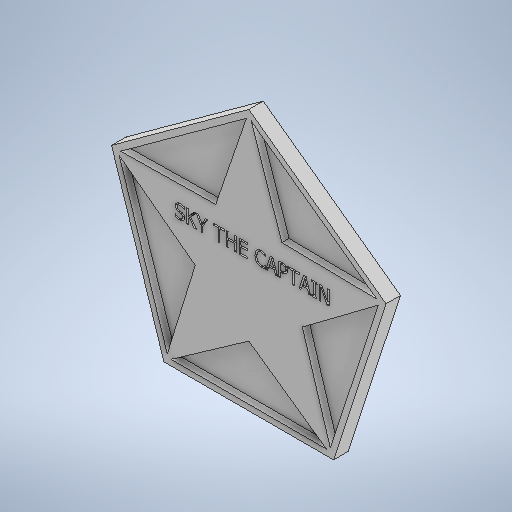
# Autodesk Inventor part: cad@24
Saved by Autodesk Inventor 2025.2 (Build 292293000, 293)
## iProperties
Created: 2025-03-15
Part Number: cad@24
Material: Generic
Document SubType Name: Modeling
Designer: spars
Density: 1 g/cm^3
Appearance: Default
Author: spars
Autodesk Inventor part; units mm, degrees
note: some values were not read from the file. Chosen so that the rebuilt part matches the saved one: direction of "Emboss1".
ref_plane "YZ Plane" through (0, 0, 0) normal (1, 0, 0) x (0, 1, 0)
ref_plane "XZ Plane" through (0, 0, 0) normal (0, 1, 0) x (-1, 0, 0)
ref_plane "XY Plane" through (0, 0, 0) normal (0, 0, 1) x (1, 0, 0)
sketch "Sketch1" plane through (0, 0, 0) normal (0, 0, 1) x (1, 0, 0)
  circle A0 centre (0, 0) radius 10 construction
  line L0 (0, 10) -> (9.5106, 3.0902)
  line L1 (9.5106, 3.0902) -> (5.8779, -8.0902)
  line L2 (5.8779, -8.0902) -> (-5.8779, -8.0902)
  line L3 (-5.8779, -8.0902) -> (-9.5106, 3.0902)
  line L4 (-9.5106, 3.0902) -> (0, 10)
  line L5 (0, 0) -> (0, -3.9)
  dimension "d0" = 20
  dimension "d1" = 3.9
  constraints: 12 end point, 2 coincident, 1 vertical, 1 vertical alignment, 13 other
  measures "d1" distance of L5.start L5.end
extrude "Extrusion1" add sketch "Sketch1" along normal blind 1
sketch "Sketch2" plane through (0, 0, 1) normal (0, 0, 1) x (1, 0, 0)
  line L0 (0.1618, 9.388) -> (8.8785, 3.0549)
  line L1 (8.9785, 2.7472) -> (5.649, -7.5)
  line L2 (5.3872, -7.6902) -> (-5.3872, -7.6902)
  line L3 (-5.649, -7.5) -> (-8.9785, 2.7472)
  line L4 (-8.8785, 3.0549) -> (-0.1618, 9.388)
  line L5 (-5.8779, -8.0902) -> (5.8779, -8.0902) projected
  line L6 (5.8779, -8.0902) -> (9.5106, 3.0902) projected
  line L7 (0, 10) -> (-9.5106, 3.0902) projected
  line L8 (9.5106, 3.0902) -> (0, 10) projected
  line L9 (-9.5106, 3.0902) -> (-5.8779, -8.0902) projected
  line L10 (0, 0) -> (0, -3.9)
  line L11 (0, -3.9) -> (-5.3872, -7.6902)
  line L12 (0, -3.9) -> (5.3872, -7.6902)
  line L13 (3.7091, -1.2052) -> (5.649, -7.5)
  line L14 (3.7091, -1.2052) -> (8.9785, 2.7472)
  line L15 (2.2924, 3.1552) -> (8.8785, 3.0549)
  line L16 (2.2924, 3.1552) -> (0.1618, 9.388)
  line L17 (-2.2924, 3.1552) -> (-0.1618, 9.388)
  line L18 (-2.2924, 3.1552) -> (-8.8785, 3.0549)
  line L19 (-3.7091, -1.2052) -> (-8.9785, 2.7472)
  line L20 (-3.7091, -1.2052) -> (-5.649, -7.5)
  point P0 (0, 9.5056)
  point P1 (9.0403, 2.9374)
  point P2 (5.5872, -7.6902)
  point P3 (-5.5872, -7.6902)
  point P4 (-9.0403, 2.9374)
  point P5 (8.8785, 3.0549)
  point P6 (-8.9785, 2.7472)
  dimension "d4" = 0.4
  dimension "d5" = 0.4
  dimension "d6" = 0.4
  dimension "d7" = 0.4
  dimension "d8" = 0.4
  dimension "d9" = 0.2
  dimension "d10" = 0.2
  dimension "d11" = 0.2
  dimension "d12" = 0.2
  dimension "d13" = 0.2
  dimension "d14" = 0.2
  dimension "d15" = 0.2
  dimension "d16" = 0.2
  dimension "d17" = 0.2
  dimension "d18" = 0.2
  dimension "d19" = 3.9
  dimension "d22" = 360
  constraints: 32 end point, 10 point on line, 1 coincident, 1 vertical, 37 other
  measures "d4" distance between parallel lines of L5 L2
  measures "d5" distance between parallel lines of L6 L1
  measures "d6" distance between parallel lines of L4 L7
  measures "d7" distance between parallel lines of L0 L8
  measures "d8" distance between parallel lines of L9 L3
  measures "d9" distance of L3.end point (-9.04, 2.937)
  measures "d10" distance of L4.start point (-9.04, 2.937)
  measures "d11" distance of L4.end point (0, 9.506)
  measures "d12" distance of L0.start point (0, 9.506)
  measures "d13" distance of L0.end point (9.04, 2.937)
  measures "d14" distance of L1.start point (9.04, 2.937)
  measures "d15" distance of L2.start point (5.587, -7.69)
  measures "d16" distance of L1.end point (5.587, -7.69)
  measures "d17" distance of L3.start point (-5.587, -7.69)
  measures "d18" distance of L2.end point (-5.587, -7.69)
  measures "d19" distance of L10.start L10.end
extrude "Extrusion2" cut sketch "Sketch2" against normal blind 0.5 contours L0 L15 L16 | L1 L13 L14 | L2 L11 L12 | L3 L19 L20 | L4 L17 L18
sketch "Sketch3" plane through (0, 0, 1) normal (0, 0, 1) x (1, 0, 0)
  line L0 (-5.1512, 1.9683) -> (5.6683, 1.9683) construction
  line L1 (5.6683, 1.9683) -> (5.6683, 0.9676) construction
  line L2 (5.6683, 0.9676) -> (-5.1512, 0.9676) construction
  line L3 (-5.1512, 0.9676) -> (-5.1512, 1.9683) construction
  spline S0 degree 2 poles (-4.7839, 0.9676) (-4.8889, 0.9676) (-5.0361, 1.0115) (-5.1011, 1.0428) knots 0 0 0 1 2 2 2
  line L4 (-5.1011, 1.0428) -> (-5.1011, 1.2041)
  line L5 (-5.1011, 1.2041) -> (-5.0917, 1.2041)
  spline S1 degree 2 poles (-5.0917, 1.2041) (-5.0282, 1.1446) (-4.8677, 1.0788) (-4.7933, 1.0788) knots 0 0 0 1 2 2 2
  spline S2 degree 2 poles (-4.7933, 1.0788) (-4.6869, 1.0788) (-4.578, 1.1673) (-4.578, 1.2401) knots 0 0 0 1 2 2 2
  spline S3 degree 2 poles (-4.578, 1.2401) (-4.578, 1.2981) (-4.6352, 1.3701) (-4.697, 1.3881) knots 0 0 0 1 2 2 2
  spline S4 degree 2 poles (-4.697, 1.3881) (-4.7417, 1.4006) (-4.816, 1.4179) (-4.8716, 1.432) knots 0 0 0 1 2 2 2
  spline S5 degree 2 poles (-4.8716, 1.432) (-4.9217, 1.4453) (-5.0008, 1.4852) (-5.0314, 1.5173) knots 0 0 0 1 2 2 2
  spline S6 degree 2 poles (-5.0314, 1.5173) (-5.0611, 1.5494) (-5.094, 1.6355) (-5.094, 1.6919) knots 0 0 0 1 2 2 2
  spline S7 degree 2 poles (-5.094, 1.6919) (-5.094, 1.8094) (-4.9108, 1.9683) (-4.7691, 1.9683) knots 0 0 0 1 2 2 2
  spline S8 degree 2 poles (-4.7691, 1.9683) (-4.6876, 1.9683) (-4.5436, 1.9362) (-4.4817, 1.9057) knots 0 0 0 1 2 2 2
  line L6 (-4.4817, 1.9057) -> (-4.4817, 1.7522)
  line L7 (-4.4817, 1.7522) -> (-4.4911, 1.7522)
  spline S9 degree 2 poles (-4.4911, 1.7522) (-4.5373, 1.7945) (-4.6814, 1.8571) (-4.7605, 1.8571) knots 0 0 0 1 2 2 2
  spline S10 degree 2 poles (-4.7605, 1.8571) (-4.8497, 1.8571) (-4.9601, 1.7733) (-4.9601, 1.7052) knots 0 0 0 1 2 2 2
  spline S11 degree 2 poles (-4.9601, 1.7052) (-4.9601, 1.6442) (-4.8951, 1.5713) (-4.8341, 1.5549) knots 0 0 0 1 2 2 2
  spline S12 degree 2 poles (-4.8341, 1.5549) (-4.7933, 1.5439) (-4.6751, 1.5157) (-4.636, 1.504) knots 0 0 0 1 2 2 2
  spline S13 degree 2 poles (-4.636, 1.504) (-4.5365, 1.4735) (-4.4441, 1.3505) (-4.4441, 1.2605) knots 0 0 0 1 2 2 2
  spline S14 degree 2 poles (-4.4441, 1.2605) (-4.4441, 1.2033) (-4.4903, 1.0937) (-4.5318, 1.0553) knots 0 0 0 1 2 2 2
  spline S15 degree 2 poles (-4.5318, 1.0553) (-4.578, 1.0131) (-4.6955, 0.9676) (-4.7839, 0.9676) knots 0 0 0 1 2 2 2
  line L8 (-3.6087, 0.9849) -> (-3.7754, 0.9849)
  line L9 (-3.7754, 0.9849) -> (-4.1286, 1.4343)
  line L10 (-4.1286, 1.4343) -> (-4.185, 1.3709)
  line L11 (-4.185, 1.3709) -> (-4.185, 0.9849)
  line L12 (-4.185, 0.9849) -> (-4.3134, 0.9849)
  line L13 (-4.3134, 0.9849) -> (-4.3134, 1.9511)
  line L14 (-4.3134, 1.9511) -> (-4.185, 1.9511)
  line L15 (-4.185, 1.9511) -> (-4.185, 1.5071)
  line L16 (-4.185, 1.5071) -> (-3.7888, 1.9511)
  line L17 (-3.7888, 1.9511) -> (-3.6322, 1.9511)
  line L18 (-3.6322, 1.9511) -> (-4.0323, 1.5197)
  line L19 (-4.0323, 1.5197) -> (-3.6087, 0.9849)
  line L20 (-2.8554, 1.9511) -> (-3.1819, 1.4124)
  line L21 (-3.1819, 1.4124) -> (-3.1819, 0.9849)
  line L22 (-3.1819, 0.9849) -> (-3.3103, 0.9849)
  line L23 (-3.3103, 0.9849) -> (-3.3103, 1.3991)
  line L24 (-3.3103, 1.3991) -> (-3.6369, 1.9511)
  line L25 (-3.6369, 1.9511) -> (-3.4943, 1.9511)
  line L26 (-3.4943, 1.9511) -> (-3.2454, 1.5259)
  line L27 (-3.2454, 1.5259) -> (-2.9917, 1.9511)
  line L28 (-2.9917, 1.9511) -> (-2.8554, 1.9511)
  line L29 (-2.1257, 0.9849) -> (-2.1257, 1.8368)
  line L30 (-2.1257, 1.8368) -> (-2.4498, 1.8368)
  line L31 (-2.4498, 1.8368) -> (-2.4498, 1.9511)
  line L32 (-2.4498, 1.9511) -> (-1.6731, 1.9511)
  line L33 (-1.6731, 1.9511) -> (-1.6731, 1.8368)
  line L34 (-1.6731, 1.8368) -> (-1.9973, 1.8368)
  line L35 (-1.9973, 1.8368) -> (-1.9973, 0.9849)
  line L36 (-1.9973, 0.9849) -> (-2.1257, 0.9849)
  line L37 (-0.8737, 0.9849) -> (-1.0021, 0.9849)
  line L38 (-1.0021, 0.9849) -> (-1.0021, 1.4578)
  line L39 (-1.0021, 1.4578) -> (-1.4468, 1.4578)
  line L40 (-1.4468, 1.4578) -> (-1.4468, 0.9849)
  line L41 (-1.4468, 0.9849) -> (-1.5752, 0.9849)
  line L42 (-1.5752, 0.9849) -> (-1.5752, 1.9511)
  line L43 (-1.5752, 1.9511) -> (-1.4468, 1.9511)
  line L44 (-1.4468, 1.9511) -> (-1.4468, 1.5721)
  line L45 (-1.4468, 1.5721) -> (-1.0021, 1.5721)
  line L46 (-1.0021, 1.5721) -> (-1.0021, 1.9511)
  line L47 (-1.0021, 1.9511) -> (-0.8737, 1.9511)
  line L48 (-0.8737, 1.9511) -> (-0.8737, 0.9849)
  line L49 (-0.6779, 0.9849) -> (-0.6779, 1.9511)
  line L50 (-0.6779, 1.9511) -> (-0.0734, 1.9511)
  line L51 (-0.0734, 1.9511) -> (-0.0734, 1.8368)
  line L52 (-0.0734, 1.8368) -> (-0.5495, 1.8368)
  line L53 (-0.5495, 1.8368) -> (-0.5495, 1.5721)
  line L54 (-0.5495, 1.5721) -> (-0.1055, 1.5721)
  line L55 (-0.1055, 1.5721) -> (-0.1055, 1.4578)
  line L56 (-0.1055, 1.4578) -> (-0.5495, 1.4578)
  line L57 (-0.5495, 1.4578) -> (-0.5495, 1.0992)
  line L58 (-0.5495, 1.0992) -> (-0.0734, 1.0992)
  line L59 (-0.0734, 1.0992) -> (-0.0734, 0.9849)
  line L60 (-0.0734, 0.9849) -> (-0.6779, 0.9849)
  spline S16 degree 2 poles (0.8599, 0.9676) (0.7659, 0.9676) (0.607, 1.0311) (0.549, 1.0945) knots 0 0 0 1 2 2 2
  spline S17 degree 2 poles (0.549, 1.0945) (0.4911, 1.1571) (0.4277, 1.345) (0.4277, 1.4672) knots 0 0 0 1 2 2 2
  spline S18 degree 2 poles (0.4277, 1.4672) (0.4277, 1.5886) (0.4895, 1.7686) (0.5483, 1.8352) knots 0 0 0 1 2 2 2
  spline S19 degree 2 poles (0.5483, 1.8352) (0.6062, 1.9002) (0.7644, 1.9683) (0.8622, 1.9683) knots 0 0 0 1 2 2 2
  spline S20 degree 2 poles (0.8622, 1.9683) (0.9108, 1.9683) (0.9961, 1.9542) (1.0321, 1.9433) knots 0 0 0 1 2 2 2
  spline S21 degree 2 poles (1.0321, 1.9433) (1.0635, 1.9331) (1.1285, 1.9041) (1.1606, 1.8869) knots 0 0 0 1 2 2 2
  line L61 (1.1606, 1.8869) -> (1.1606, 1.7318)
  line L62 (1.1606, 1.7318) -> (1.1504, 1.7318)
  spline S22 degree 2 poles (1.1504, 1.7318) (1.1332, 1.7475) (1.0799, 1.7914) (1.0415, 1.8125) knots 0 0 0 1 2 2 2
  spline S23 degree 2 poles (1.0415, 1.8125) (1.0047, 1.8329) (0.9178, 1.8587) (0.8615, 1.8587) knots 0 0 0 1 2 2 2
  spline S24 degree 2 poles (0.8615, 1.8587) (0.7996, 1.8587) (0.6892, 1.8078) (0.6477, 1.7593) knots 0 0 0 1 2 2 2
  spline S25 degree 2 poles (0.6477, 1.7593) (0.607, 1.7099) (0.5616, 1.5604) (0.5616, 1.4672) knots 0 0 0 1 2 2 2
  spline S26 degree 2 poles (0.5616, 1.4672) (0.5616, 1.3678) (0.6093, 1.2245) (0.6508, 1.1751) knots 0 0 0 1 2 2 2
  spline S27 degree 2 poles (0.6508, 1.1751) (0.6915, 1.1274) (0.8004, 1.0788) (0.8615, 1.0788) knots 0 0 0 1 2 2 2
  spline S28 degree 2 poles (0.8615, 1.0788) (0.917, 1.0788) (1.0118, 1.1062) (1.0486, 1.1266) knots 0 0 0 1 2 2 2
  spline S29 degree 2 poles (1.0486, 1.1266) (1.0838, 1.147) (1.1363, 1.1892) (1.1512, 1.2041) knots 0 0 0 1 2 2 2
  line L63 (1.1512, 1.2041) -> (1.1606, 1.2041)
  line L64 (1.1606, 1.2041) -> (1.1606, 1.0506)
  spline S30 degree 2 poles (1.1606, 1.0506) (1.1285, 1.0358) (1.0721, 1.0084) (1.0321, 0.9958) knots 0 0 0 1 2 2 2
  spline S31 degree 2 poles (1.0321, 0.9958) (0.9899, 0.9817) (0.9178, 0.9676) (0.8599, 0.9676) knots 0 0 0 1 2 2 2
  line L65 (1.1762, 0.9849) -> (1.5019, 1.9511)
  line L66 (1.5019, 1.9511) -> (1.6601, 1.9511)
  line L67 (1.6601, 1.9511) -> (1.9858, 0.9849)
  line L68 (1.9858, 0.9849) -> (1.8504, 0.9849)
  line L69 (1.8504, 0.9849) -> (1.7627, 1.255)
  line L70 (1.7627, 1.255) -> (1.3939, 1.255)
  line L71 (1.3939, 1.255) -> (1.3062, 0.9849)
  line L72 (1.3062, 0.9849) -> (1.1762, 0.9849)
  line L73 (1.7274, 1.3646) -> (1.5779, 1.8195)
  line L74 (1.5779, 1.8195) -> (1.4291, 1.3646)
  line L75 (1.4291, 1.3646) -> (1.7274, 1.3646)
  spline S32 degree 2 poles (2.6882, 1.6598) (2.6882, 1.5972) (2.6436, 1.4844) (2.6036, 1.4453) knots 0 0 0 1 2 2 2
  spline S33 degree 2 poles (2.6036, 1.4453) (2.5535, 1.3959) (2.418, 1.345) (2.3147, 1.345) knots 0 0 0 1 2 2 2
  line L76 (2.3147, 1.345) -> (2.2059, 1.345)
  line L77 (2.2059, 1.345) -> (2.2059, 0.9849)
  line L78 (2.2059, 0.9849) -> (2.0774, 0.9849)
  line L79 (2.0774, 0.9849) -> (2.0774, 1.9511)
  line L80 (2.0774, 1.9511) -> (2.3202, 1.9511)
  spline S34 degree 2 poles (2.3202, 1.9511) (2.4063, 1.9511) (2.5269, 1.9229) (2.5731, 1.8908) knots 0 0 0 1 2 2 2
  spline S35 degree 2 poles (2.5731, 1.8908) (2.6271, 1.854) (2.6882, 1.7405) (2.6882, 1.6598) knots 0 0 0 1 2 2 2
  spline S36 degree 2 poles (2.5543, 1.6559) (2.5543, 1.706) (2.5198, 1.7796) (2.4846, 1.8031) knots 0 0 0 1 2 2 2
  spline S37 degree 2 poles (2.4846, 1.8031) (2.4541, 1.8235) (2.3726, 1.8399) (2.3123, 1.8399) knots 0 0 0 1 2 2 2
  line L81 (2.3123, 1.8399) -> (2.2059, 1.8399)
  line L82 (2.2059, 1.8399) -> (2.2059, 1.4547)
  line L83 (2.2059, 1.4547) -> (2.2936, 1.4547)
  spline S38 degree 2 poles (2.2936, 1.4547) (2.3719, 1.4547) (2.4682, 1.4797) (2.4995, 1.5126) knots 0 0 0 1 2 2 2
  spline S39 degree 2 poles (2.4995, 1.5126) (2.5285, 1.5416) (2.5543, 1.6097) (2.5543, 1.6559) knots 0 0 0 1 2 2 2
  line L84 (3.0358, 0.9849) -> (3.0358, 1.8368)
  line L85 (3.0358, 1.8368) -> (2.7117, 1.8368)
  line L86 (2.7117, 1.8368) -> (2.7117, 1.9511)
  line L87 (2.7117, 1.9511) -> (3.4884, 1.9511)
  line L88 (3.4884, 1.9511) -> (3.4884, 1.8368)
  line L89 (3.4884, 1.8368) -> (3.1642, 1.8368)
  line L90 (3.1642, 1.8368) -> (3.1642, 0.9849)
  line L91 (3.1642, 0.9849) -> (3.0358, 0.9849)
  line L92 (3.4821, 0.9849) -> (3.8079, 1.9511)
  line L93 (3.8079, 1.9511) -> (3.966, 1.9511)
  line L94 (3.966, 1.9511) -> (4.2918, 0.9849)
  line L95 (4.2918, 0.9849) -> (4.1563, 0.9849)
  line L96 (4.1563, 0.9849) -> (4.0686, 1.255)
  line L97 (4.0686, 1.255) -> (3.6998, 1.255)
  line L98 (3.6998, 1.255) -> (3.6121, 0.9849)
  line L99 (3.6121, 0.9849) -> (3.4821, 0.9849)
  line L100 (4.0334, 1.3646) -> (3.8838, 1.8195)
  line L101 (3.8838, 1.8195) -> (3.735, 1.3646)
  line L102 (3.735, 1.3646) -> (4.0334, 1.3646)
  line L103 (4.7201, 0.9849) -> (4.3458, 0.9849)
  line L104 (4.3458, 0.9849) -> (4.3458, 1.0835)
  line L105 (4.3458, 1.0835) -> (4.4687, 1.0835)
  line L106 (4.4687, 1.0835) -> (4.4687, 1.8524)
  line L107 (4.4687, 1.8524) -> (4.3458, 1.8524)
  line L108 (4.3458, 1.8524) -> (4.3458, 1.9511)
  line L109 (4.3458, 1.9511) -> (4.7201, 1.9511)
  line L110 (4.7201, 1.9511) -> (4.7201, 1.8524)
  line L111 (4.7201, 1.8524) -> (4.5971, 1.8524)
  line L112 (4.5971, 1.8524) -> (4.5971, 1.0835)
  line L113 (4.5971, 1.0835) -> (4.7201, 1.0835)
  line L114 (4.7201, 1.0835) -> (4.7201, 0.9849)
  line L115 (5.5704, 0.9849) -> (5.4263, 0.9849)
  line L116 (5.4263, 0.9849) -> (4.9988, 1.818)
  line L117 (4.9988, 1.818) -> (4.9988, 0.9849)
  line L118 (4.9988, 0.9849) -> (4.879, 0.9849)
  line L119 (4.879, 0.9849) -> (4.879, 1.9511)
  line L120 (4.879, 1.9511) -> (5.0614, 1.9511)
  line L121 (5.0614, 1.9511) -> (5.4506, 1.1861)
  line L122 (5.4506, 1.1861) -> (5.4506, 1.9511)
  line L123 (5.4506, 1.9511) -> (5.5704, 1.9511)
  line L124 (5.5704, 1.9511) -> (5.5704, 0.9849)
  point P0 (0, 0)
  constraints: 2 other
emboss "Emboss1" sketch "Sketch3" operation cut depth 0.5 direction (0, 0, -1)
equation "\"d10\" = d9"
equation "\"d11\" = d9"
equation "\"d12\" = d11"
equation "\"d13\" = d9"
equation "\"d14\" = d13"
equation "\"d15\" = d9"
equation "\"d16\" = d15"
equation "\"d17\" = d9"
equation "\"d18\" = d17"
body "Solid1"
